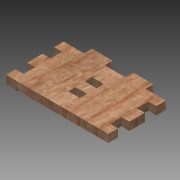
# Autodesk Inventor part: drive_support_side
Saved by Autodesk Inventor 2015 (Build 190159000, 159)
## iProperties
Created: 2013-12-24
Part Number: drive_support_side
Material: Wood (Birch)
Document SubType Name: Modeling
Designer: aoki
Density: 1 g/cm^3
Appearance: Birch - Natural Polished
d0: 71.000 mm
d1: 40.000 mm
d2: 5.500 mm
d3: 0.00 deg
Author: aoki
Autodesk Inventor part; units mm, degrees
ref_plane "YZ Plane" through (0, 0, 0) normal (1, 0, 0) x (0, 1, 0)
ref_plane "XZ Plane" through (0, 0, 0) normal (0, 1, 0) x (-1, 0, 0)
ref_plane "XY Plane" through (0, 0, 0) normal (0, 0, 1) x (1, 0, 0)
sketch "Block1" plane through (0, 0, 0) normal (0, 0, 1) x (1, 0, 0)
  line L0 (-23.62, 29.22) -> (-7.58, 29.22)
  line L1 (-7.58, 29.22) -> (-7.58, 20.22)
  line L2 (-7.58, 20.22) -> (7.58, 20.22)
  line L3 (7.58, 20.22) -> (7.58, 29.22)
  line L4 (7.58, 29.22) -> (23.62, 29.22)
  line L5 (23.62, 29.22) -> (23.62, 20.22)
  line L6 (23.62, 20.22) -> (39.22, 20.22)
  line L7 (39.22, 20.22) -> (39.22, 13.1133)
  line L8 (39.22, 13.1133) -> (30.22, 13.1133)
  line L9 (30.22, 13.1133) -> (30.22, 5.5533)
  line L10 (30.22, 5.5533) -> (39.22, 5.5533)
  line L11 (39.22, 5.5533) -> (39.22, -5.5533)
  line L12 (39.22, -5.5533) -> (30.22, -5.5533)
  line L13 (30.22, -5.5533) -> (30.22, -13.1133)
  line L14 (30.22, -13.1133) -> (39.22, -13.1133)
  line L15 (39.22, -13.1133) -> (39.22, -20.22)
  line L16 (39.22, -20.22) -> (-39.22, -20.22)
  line L17 (-39.22, -20.22) -> (-39.22, -13.1133)
  line L18 (-39.22, -13.1133) -> (-30.22, -13.1133)
  line L19 (-30.22, -13.1133) -> (-30.22, -5.5533)
  line L20 (-30.22, -5.5533) -> (-39.22, -5.5533)
  line L21 (-39.22, -5.5533) -> (-39.22, 5.5533)
  line L22 (-39.22, 5.5533) -> (-30.22, 5.5533)
  line L23 (-30.22, 5.5533) -> (-30.22, 13.1133)
  line L24 (-30.22, 13.1133) -> (-39.22, 13.1133)
  line L25 (-39.22, 13.1133) -> (-39.22, 20.22)
  line L26 (-39.22, 20.22) -> (-23.62, 20.22)
  line L27 (-23.62, 20.22) -> (-23.62, 29.22)
  line L28 (4.22, 8.55) -> (4.22, 3.11)
  line L29 (4.22, 3.11) -> (-4.22, 3.11)
  line L30 (-4.22, 3.11) -> (-4.22, 8.55)
  line L31 (-4.22, 8.55) -> (4.22, 8.55)
  line L32 (4.22, -3.11) -> (4.22, -8.55)
  line L33 (4.22, -8.55) -> (-4.22, -8.55)
  line L34 (-4.22, -8.55) -> (-4.22, -3.11)
  line L35 (-4.22, -3.11) -> (4.22, -3.11)
  point P0 (0, 5.4933)
sketch "Block2" plane through (0, 0, 0) normal (0, 0, 1) x (1, 0, 0)
  line L0 (-23.5, 29.1) -> (-7.7, 29.1)
  line L1 (-7.7, 29.1) -> (-7.7, 20.1)
  line L2 (-7.7, 20.1) -> (7.7, 20.1)
  line L3 (7.7, 20.1) -> (7.7, 29.1)
  line L4 (7.7, 29.1) -> (23.5, 29.1)
  line L5 (23.5, 29.1) -> (23.5, 20.1)
  line L6 (23.5, 20.1) -> (39.1, 20.1)
  line L7 (39.1, 20.1) -> (39.1, 13.2333)
  line L8 (39.1, 13.2333) -> (30.1, 13.2333)
  line L9 (30.1, 13.2333) -> (30.1, 5.4333)
  line L10 (30.1, 5.4333) -> (39.1, 5.4333)
  line L11 (39.1, 5.4333) -> (39.1, -5.4333)
  line L12 (39.1, -5.4333) -> (30.1, -5.4333)
  line L13 (30.1, -5.4333) -> (30.1, -13.2333)
  line L14 (30.1, -13.2333) -> (39.1, -13.2333)
  line L15 (39.1, -13.2333) -> (39.1, -20.1)
  line L16 (39.1, -20.1) -> (-39.1, -20.1)
  line L17 (-39.1, -20.1) -> (-39.1, -13.2333)
  line L18 (-39.1, -13.2333) -> (-30.1, -13.2333)
  line L19 (-30.1, -13.2333) -> (-30.1, -5.4333)
  line L20 (-30.1, -5.4333) -> (-39.1, -5.4333)
  line L21 (-39.1, -5.4333) -> (-39.1, 5.4333)
  line L22 (-39.1, 5.4333) -> (-30.1, 5.4333)
  line L23 (-30.1, 5.4333) -> (-30.1, 13.2333)
  line L24 (-30.1, 13.2333) -> (-39.1, 13.2333)
  line L25 (-39.1, 13.2333) -> (-39.1, 20.1)
  line L26 (-39.1, 20.1) -> (-23.5, 20.1)
  line L27 (-23.5, 20.1) -> (-23.5, 29.1)
  line L28 (4.1, 8.43) -> (4.1, 3.23)
  line L29 (4.1, 3.23) -> (-4.1, 3.23)
  line L30 (-4.1, 3.23) -> (-4.1, 8.43)
  line L31 (-4.1, 8.43) -> (4.1, 8.43)
  line L32 (4.1, -3.23) -> (4.1, -8.43)
  line L33 (4.1, -8.43) -> (-4.1, -8.43)
  line L34 (-4.1, -8.43) -> (-4.1, -3.23)
  line L35 (-4.1, -3.23) -> (4.1, -3.23)
  point P0 (0, 5.4667)
sketch "Block3" plane through (0, 0, 0) normal (0, 0, 1) x (1, 0, 0)
  line L0 (7.6, 29.2) -> (23.6, 29.2)
  line L1 (23.6, 29.2) -> (23.6, 20.2)
  line L2 (23.6, 20.2) -> (39.2, 20.2)
  line L3 (39.2, 20.2) -> (39.2, 13.1333)
  line L4 (39.2, 13.1333) -> (30.2, 13.1333)
  line L5 (30.2, 13.1333) -> (30.2, 5.5333)
  line L6 (30.2, 5.5333) -> (39.2, 5.5333)
  line L7 (39.2, 5.5333) -> (39.2, -5.5333)
  line L8 (39.2, -5.5333) -> (30.2, -5.5333)
  line L9 (30.2, -5.5333) -> (30.2, -13.1333)
  line L10 (30.2, -13.1333) -> (39.2, -13.1333)
  line L11 (39.2, -13.1333) -> (39.2, -20.2)
  line L12 (39.2, -20.2) -> (-39.2, -20.2)
  line L13 (-39.2, -20.2) -> (-39.2, -13.1333)
  line L14 (-39.2, -13.1333) -> (-30.2, -13.1333)
  line L15 (-30.2, -13.1333) -> (-30.2, -5.5333)
  line L16 (-30.2, -5.5333) -> (-39.2, -5.5333)
  line L17 (-39.2, -5.5333) -> (-39.2, 5.5333)
  line L18 (-39.2, 5.5333) -> (-30.2, 5.5333)
  line L19 (-30.2, 5.5333) -> (-30.2, 13.1333)
  line L20 (-30.2, 13.1333) -> (-39.2, 13.1333)
  line L21 (-39.2, 13.1333) -> (-39.2, 20.2)
  line L22 (-39.2, 20.2) -> (-23.6, 20.2)
  line L23 (-23.6, 20.2) -> (-23.6, 29.2)
  line L24 (-23.6, 29.2) -> (-7.6, 29.2)
  line L25 (-7.6, 29.2) -> (-7.6, 20.2)
  line L26 (-7.6, 20.2) -> (7.6, 20.2)
  line L27 (7.6, 20.2) -> (7.6, 29.2)
  line L28 (4.2, 8.53) -> (4.2, 3.13)
  line L29 (4.2, 3.13) -> (-4.2, 3.13)
  line L30 (-4.2, 3.13) -> (-4.2, 8.53)
  line L31 (-4.2, 8.53) -> (4.2, 8.53)
  line L32 (4.2, -3.13) -> (4.2, -8.53)
  line L33 (4.2, -8.53) -> (-4.2, -8.53)
  line L34 (-4.2, -8.53) -> (-4.2, -3.13)
  line L35 (-4.2, -3.13) -> (4.2, -3.13)
  point P0 (0, 5.4889)
sketch "Block4" plane through (0, 0, 0) normal (0, 0, 1) x (1, 0, 0)
  line L0 (7.7, 29.1) -> (23.5, 29.1)
  line L1 (23.5, 29.1) -> (23.5, 20.1)
  line L2 (23.5, 20.1) -> (39.1, 20.1)
  line L3 (39.1, 20.1) -> (39.1, 13.2333)
  line L4 (39.1, 13.2333) -> (30.1, 13.2333)
  line L5 (30.1, 13.2333) -> (30.1, 5.4333)
  line L6 (30.1, 5.4333) -> (39.1, 5.4333)
  line L7 (39.1, 5.4333) -> (39.1, -5.4333)
  line L8 (39.1, -5.4333) -> (30.1, -5.4333)
  line L9 (30.1, -5.4333) -> (30.1, -13.2333)
  line L10 (30.1, -13.2333) -> (39.1, -13.2333)
  line L11 (39.1, -13.2333) -> (39.1, -20.1)
  line L12 (39.1, -20.1) -> (-39.1, -20.1)
  line L13 (-39.1, -20.1) -> (-39.1, -13.2333)
  line L14 (-39.1, -13.2333) -> (-30.1, -13.2333)
  line L15 (-30.1, -13.2333) -> (-30.1, -5.4333)
  line L16 (-30.1, -5.4333) -> (-39.1, -5.4333)
  line L17 (-39.1, -5.4333) -> (-39.1, 5.4333)
  line L18 (-39.1, 5.4333) -> (-30.1, 5.4333)
  line L19 (-30.1, 5.4333) -> (-30.1, 13.2333)
  line L20 (-30.1, 13.2333) -> (-39.1, 13.2333)
  line L21 (-39.1, 13.2333) -> (-39.1, 20.1)
  line L22 (-39.1, 20.1) -> (-23.5, 20.1)
  line L23 (-23.5, 20.1) -> (-23.5, 29.1)
  line L24 (-23.5, 29.1) -> (-7.7, 29.1)
  line L25 (-7.7, 29.1) -> (-7.7, 20.1)
  line L26 (-7.7, 20.1) -> (7.7, 20.1)
  line L27 (7.7, 20.1) -> (7.7, 29.1)
  line L28 (4.1, 8.43) -> (4.1, 3.23)
  line L29 (4.1, 3.23) -> (-4.1, 3.23)
  line L30 (-4.1, 3.23) -> (-4.1, 8.43)
  line L31 (-4.1, 8.43) -> (4.1, 8.43)
  line L32 (4.1, -3.23) -> (4.1, -8.43)
  line L33 (4.1, -8.43) -> (-4.1, -8.43)
  line L34 (-4.1, -8.43) -> (-4.1, -3.23)
  line L35 (-4.1, -3.23) -> (4.1, -3.23)
  point P0 (0, 5.4667)
sketch "Block5" plane through (0, 0, 0) normal (0, 0, 1) x (1, 0, 0)
  line L0 (-21.38, 25.58) -> (-7.02, 25.58)
  line L1 (-7.02, 25.58) -> (-7.02, 20.08)
  line L2 (-7.02, 20.08) -> (7.02, 20.08)
  line L3 (7.02, 20.08) -> (7.02, 25.58)
  line L4 (7.02, 25.58) -> (21.38, 25.58)
  line L5 (21.38, 25.58) -> (21.38, 20.08)
  line L6 (21.38, 20.08) -> (35.58, 20.08)
  line L7 (35.58, 20.08) -> (35.58, 13.2533)
  line L8 (35.58, 13.2533) -> (30.08, 13.2533)
  line L9 (30.08, 13.2533) -> (30.08, 5.4133)
  line L10 (30.08, 5.4133) -> (35.58, 5.4133)
  line L11 (35.58, 5.4133) -> (35.58, -5.4133)
  line L12 (35.58, -5.4133) -> (30.08, -5.4133)
  line L13 (30.08, -5.4133) -> (30.08, -13.2533)
  line L14 (30.08, -13.2533) -> (35.58, -13.2533)
  line L15 (35.58, -13.2533) -> (35.58, -20.08)
  line L16 (35.58, -20.08) -> (-35.58, -20.08)
  line L17 (-35.58, -20.08) -> (-35.58, -13.2533)
  line L18 (-35.58, -13.2533) -> (-30.08, -13.2533)
  line L19 (-30.08, -13.2533) -> (-30.08, -5.4133)
  line L20 (-30.08, -5.4133) -> (-35.58, -5.4133)
  line L21 (-35.58, -5.4133) -> (-35.58, 5.4133)
  line L22 (-35.58, 5.4133) -> (-30.08, 5.4133)
  line L23 (-30.08, 5.4133) -> (-30.08, 13.2533)
  line L24 (-30.08, 13.2533) -> (-35.58, 13.2533)
  line L25 (-35.58, 13.2533) -> (-35.58, 20.08)
  line L26 (-35.58, 20.08) -> (-21.38, 20.08)
  line L27 (-21.38, 20.08) -> (-21.38, 25.58)
  line L28 (4.08, 8.41) -> (4.08, 3.25)
  line L29 (4.08, 3.25) -> (-4.08, 3.25)
  line L30 (-4.08, 3.25) -> (-4.08, 8.41)
  line L31 (-4.08, 8.41) -> (4.08, 8.41)
  line L32 (4.08, -3.25) -> (4.08, -8.41)
  line L33 (4.08, -8.41) -> (-4.08, -8.41)
  line L34 (-4.08, -8.41) -> (-4.08, -3.25)
  line L35 (-4.08, -3.25) -> (4.08, -3.25)
  point P0 (0, 5.0733)
sketch "Sketch1" plane through (0, 0, 0) normal (0, 0, 1) x (1, 0, 0)
  line L0 (35.5, -20) -> (-35.5, -20)
  line L1 (-35.5, -20) -> (-35.5, 20)
  line L2 (-35.5, 20) -> (35.5, 20)
  line L3 (35.5, 20) -> (35.5, -20)
  line L4 (35.5, -20) -> (-35.5, 20) construction
  line L5 (-35.5, -20) -> (35.5, 20) construction
  point P0 (0, 0)
  point P1 (0, 0)
  dimension "d0" = 71
  dimension "d1" = 40
  constraints: 12 end point, 2 midpoint, 2 parallel, 1 coincident, 1 horizontal, 1 perpendicular
  measures "d0" distance of L1.end L2.end
  measures "d1" distance of L0.end L1.end
extrude "Extrusion1" add sketch "Sketch1" against normal blind 5.5
sketch "Sketch3" plane through (0, 0, 0) normal (0, 0, 1) x (1, 0, 0)
  line L0 (-35.5, 20) -> (35.5, 20) projected
  line L1 (-35.5, -20) -> (-35.5, 20) projected
  line L2 (-35.5, 13.3333) -> (-30, 13.3333)
  line L3 (-30, 13.3333) -> (-30, 5.3333)
  line L4 (-30, 5.3333) -> (-35.5, 5.3333)
  line L5 (-35.5, 13.3333) -> (-35.5, 5.3333)
  line L6 (-161.1974, 0) -> (72.4829, 0) projected
  line L7 (0, -29.94) -> (0, 38.94) projected
  line L8 (35.5, 13.3333) -> (30, 13.3333)
  line L9 (30, 13.3333) -> (30, 5.3333)
  line L10 (30, 5.3333) -> (35.5, 5.3333)
  line L11 (35.5, 13.3333) -> (35.5, 5.3333)
  line L12 (-35.5, -13.3333) -> (-30, -13.3333)
  line L13 (-30, -13.3333) -> (-30, -5.3333)
  line L14 (-30, -5.3333) -> (-35.5, -5.3333)
  line L15 (-35.5, -13.3333) -> (-35.5, -5.3333)
  line L16 (30, -13.3333) -> (30, -5.3333)
  line L17 (35.5, -13.3333) -> (35.5, -5.3333)
  line L18 (30, -5.3333) -> (35.5, -5.3333)
  line L19 (35.5, -13.3333) -> (30, -13.3333)
  point P0 (0, 0)
  dimension "d16" = 5.5
  dimension "d17" = 8
  dimension "d18" = 6.6667
  constraints: 32 end point, 12 symmetric about line, 2 perpendicular, 2 point on line, 1 collinear, 1 parallel
  measures "d16" distance of L2.start L2.end
  measures "d17" distance of L2.end L3.end
  measures "d18" distance between parallel lines of L0 L2
sketch "Sketch4" plane through (0, 0, 0) normal (0, 0, 1) x (1, 0, 0)
  line L0 (4, -8.33) -> (-4, -8.33)
  line L1 (-4, -8.33) -> (-4, -3.33)
  line L2 (-4, -3.33) -> (4, -3.33)
  line L3 (4, -3.33) -> (4, -8.33)
  line L4 (4, -8.33) -> (-4, -3.33) construction
  line L5 (-4, -8.33) -> (4, -3.33) construction
  line L6 (-161.1974, 0) -> (72.4829, 0) projected
  line L7 (4, 8.33) -> (-4, 8.33)
  line L8 (-4, 8.33) -> (-4, 3.33)
  line L9 (-4, 3.33) -> (4, 3.33)
  line L10 (4, 3.33) -> (4, 8.33)
  line L11 (4, 8.33) -> (-4, 3.33) construction
  line L12 (-4, 8.33) -> (4, 3.33) construction
  point P0 (0, -5.83)
  point P1 (0, 5.83)
  dimension "d25" = 8
  dimension "d26" = 5
  dimension "d27" = 3.33
  constraints: 24 end point, 5 symmetric about line, 4 midpoint, 2 parallel, 1 horizontal, 1 perpendicular
  measures "d25" distance of L1.end L2.end
  measures "d26" distance of L0.end L1.end
  measures "d27" distance between parallel lines of L6 L2
extrude "Extrusion4" cut sketch "Sketch4" against normal through all
extrude "Extrusion5" cut sketch "Sketch3" against normal through all contours L2 L3 L4 L1 | L1 L14 L13 L12 | L11 L10 L9 L8 | L16 L18 L17 L19
sketch "Sketch5" plane through (0, 0, 0) normal (0, 0, 1) x (1, 0, 0)
  line L0 (-35.5, 20) -> (35.5, 20) projected
  line L1 (-21.3, 20) -> (-7.1, 20)
  line L2 (-7.1, 20) -> (-7.1, 25.5)
  line L3 (-7.1, 25.5) -> (-21.3, 25.5)
  line L4 (-21.3, 25.5) -> (-21.3, 20)
  line L5 (0, -29.94) -> (0, 38.94) projected
  line L6 (21.3, 20) -> (7.1, 20)
  line L7 (7.1, 20) -> (7.1, 25.5)
  line L8 (7.1, 25.5) -> (21.3, 25.5)
  line L9 (21.3, 25.5) -> (21.3, 20)
  point P0 (0, 0)
  dimension "d32" = 14.2
  dimension "d33" = 14.2
  dimension "d34" = 5.5
  constraints: 16 end point, 4 symmetric about line, 2 parallel, 1 horizontal, 1 perpendicular, 1 point on line
  measures "d32" distance from line of L0.start L4
  measures "d33" distance of L2.end L3.end
  measures "d34" distance of L1.end L2.end
extrude "Extrusion6" add sketch "Sketch5" against normal blind 5.5
equation "\"d2\" = Wt"
equation "\"d16\" = Wt"
equation "\"d17\" = 0.2 * d1"
equation "\"d18\" = 0.166667 * d1"
equation "\"d32\" = 0.2 * d0"
equation "\"d33\" = 0.2 * d0"
equation "\"d34\" = Wt"
equation "\"d35\" = Wt"
equation "\"testKerf1\" = 1"
equation "\"Wt\" = 5.5"
body "Solid1"
